Autodesk Inventor part; units mm, degrees
(part 3 of 3)
  line L1481 (57.9743, 33.8467) -> (57.6371, 34.1533)
  line L1482 (57.6371, 34.1533) -> (57.3304, 34.4906)
  line L1483 (57.3304, 34.4906) -> (57.0572, 34.8563)
  line L1484 (57.0572, 34.8563) -> (56.8192, 35.2478)
  line L1485 (56.8192, 35.2478) -> (56.6194, 35.6631)
  line L1486 (56.6194, 35.6631) -> (56.4595, 36.0994)
  line L1487 (56.4595, 36.0994) -> (56.3424, 36.5547)
  line L1488 (56.3424, 36.5547) -> (56.2704, 37.0263)
  line L1489 (56.2704, 37.0263) -> (56.2459, 37.5119)
  line L1490 (-65.7501, 37.5) -> (-65.7256, 37.9856)
  line L1491 (-65.7256, 37.9856) -> (-65.6536, 38.4573)
  line L1492 (-65.6536, 38.4573) -> (-65.5365, 38.9125)
  line L1493 (-65.5365, 38.9125) -> (-65.3768, 39.3488)
  line L1494 (-65.3768, 39.3488) -> (-65.1768, 39.7642)
  line L1495 (-65.1768, 39.7642) -> (-64.9389, 40.1557)
  line L1496 (-64.9389, 40.1557) -> (-64.6654, 40.5214)
  line L1497 (-64.6654, 40.5214) -> (-64.3588, 40.8588)
  line L1498 (-64.3588, 40.8588) -> (-64.0215, 41.1653)
  line L1499 (-64.0215, 41.1653) -> (-63.6558, 41.4388)
  line L1500 (-63.6558, 41.4388) -> (-63.2643, 41.6767)
  line L1501 (-63.2643, 41.6767) -> (-62.849, 41.8767)
  line L1502 (-62.849, 41.8767) -> (-62.4126, 42.0364)
  line L1503 (-62.4126, 42.0364) -> (-61.9574, 42.1535)
  line L1504 (-61.9574, 42.1535) -> (-61.4857, 42.2255)
  line L1505 (-61.4857, 42.2255) -> (-61.0002, 42.25)
  line L1506 (-61.0002, 42.25) -> (-60.5144, 42.2255)
  line L1507 (-60.5144, 42.2255) -> (-60.0428, 42.1535)
  line L1508 (-60.0428, 42.1535) -> (-59.5877, 42.0364)
  line L1509 (-59.5877, 42.0364) -> (-59.1512, 41.8767)
  line L1510 (-59.1512, 41.8767) -> (-58.736, 41.6767)
  line L1511 (-58.736, 41.6767) -> (-58.3443, 41.4388)
  line L1512 (-58.3443, 41.4388) -> (-57.9786, 41.1653)
  line L1513 (-57.9786, 41.1653) -> (-57.6414, 40.8588)
  line L1514 (-57.6414, 40.8588) -> (-57.3347, 40.5214)
  line L1515 (-57.3347, 40.5214) -> (-57.0614, 40.1557)
  line L1516 (-57.0614, 40.1557) -> (-56.8233, 39.7642)
  line L1517 (-56.8233, 39.7642) -> (-56.6233, 39.3488)
  line L1518 (-56.6233, 39.3488) -> (-56.4637, 38.9125)
  line L1519 (-56.4637, 38.9125) -> (-56.3465, 38.4573)
  line L1520 (-56.3465, 38.4573) -> (-56.2747, 37.9856)
  line L1521 (-56.2747, 37.9856) -> (-56.2501, 37.5)
  line L1522 (-56.2501, 37.5) -> (-56.2747, 37.0143)
  line L1523 (-56.2747, 37.0143) -> (-56.3465, 36.5426)
  line L1524 (-56.3465, 36.5426) -> (-56.4637, 36.0875)
  line L1525 (-56.4637, 36.0875) -> (-56.6233, 35.6511)
  line L1526 (-56.6233, 35.6511) -> (-56.8233, 35.2359)
  line L1527 (-56.8233, 35.2359) -> (-57.0614, 34.8442)
  line L1528 (-57.0614, 34.8442) -> (-57.3347, 34.4785)
  line L1529 (-57.3347, 34.4785) -> (-57.6414, 34.1412)
  line L1530 (-57.6414, 34.1412) -> (-57.9786, 33.8346)
  line L1531 (-57.9786, 33.8346) -> (-58.3443, 33.5613)
  line L1532 (-58.3443, 33.5613) -> (-58.736, 33.3234)
  line L1533 (-58.736, 33.3234) -> (-59.1512, 33.1232)
  line L1534 (-59.1512, 33.1232) -> (-59.5877, 32.9635)
  line L1535 (-59.5877, 32.9635) -> (-60.0428, 32.8466)
  line L1536 (-60.0428, 32.8466) -> (-60.5144, 32.7746)
  line L1537 (-60.5144, 32.7746) -> (-61.0002, 32.7499)
  line L1538 (-61.0002, 32.7499) -> (-61.4857, 32.7746)
  line L1539 (-61.4857, 32.7746) -> (-61.9574, 32.8466)
  line L1540 (-61.9574, 32.8466) -> (-62.4126, 32.9635)
  line L1541 (-62.4126, 32.9635) -> (-62.849, 33.1232)
  line L1542 (-62.849, 33.1232) -> (-63.2643, 33.3234)
  line L1543 (-63.2643, 33.3234) -> (-63.6558, 33.5613)
  line L1544 (-63.6558, 33.5613) -> (-64.0215, 33.8346)
  line L1545 (-64.0215, 33.8346) -> (-64.3588, 34.1412)
  line L1546 (-64.3588, 34.1412) -> (-64.6654, 34.4785)
  line L1547 (-64.6654, 34.4785) -> (-64.9389, 34.8442)
  line L1548 (-64.9389, 34.8442) -> (-65.1768, 35.2359)
  line L1549 (-65.1768, 35.2359) -> (-65.3768, 35.6511)
  line L1550 (-65.3768, 35.6511) -> (-65.5365, 36.0875)
  line L1551 (-65.5365, 36.0875) -> (-65.6536, 36.5426)
  line L1552 (-65.6536, 36.5426) -> (-65.7256, 37.0143)
  line L1553 (-65.7256, 37.0143) -> (-65.7501, 37.5)
  line L1554 (58.9, 61.0109) -> (58.9107, 61.2257)
  line L1555 (58.9107, 61.2257) -> (58.9427, 61.4341)
  line L1556 (58.9427, 61.4341) -> (58.9944, 61.6355)
  line L1557 (58.9944, 61.6355) -> (59.065, 61.8284)
  line L1558 (59.065, 61.8284) -> (59.1532, 62.0121)
  line L1559 (59.1532, 62.0121) -> (59.2587, 62.1852)
  line L1560 (59.2587, 62.1852) -> (59.3796, 62.3468)
  line L1561 (59.3796, 62.3468) -> (59.515, 62.4959)
  line L1562 (59.515, 62.4959) -> (59.6641, 62.6315)
  line L1563 (59.6641, 62.6315) -> (59.8257, 62.7524)
  line L1564 (59.8257, 62.7524) -> (59.999, 62.8575)
  line L1565 (59.999, 62.8575) -> (60.1826, 62.946)
  line L1566 (60.1826, 62.946) -> (60.3756, 63.0167)
  line L1567 (60.3756, 63.0167) -> (60.5768, 63.0683)
  line L1568 (60.5768, 63.0683) -> (60.7852, 63.1002)
  line L1569 (60.7852, 63.1002) -> (60.9998, 63.111)
  line L1570 (60.9998, 63.111) -> (61.2148, 63.1002)
  line L1571 (61.2148, 63.1002) -> (61.4232, 63.0683)
  line L1572 (61.4232, 63.0683) -> (61.6244, 63.0167)
  line L1573 (61.6244, 63.0167) -> (61.8173, 62.946)
  line L1574 (61.8173, 62.946) -> (62.001, 62.8575)
  line L1575 (62.001, 62.8575) -> (62.1739, 62.7524)
  line L1576 (62.1739, 62.7524) -> (62.3358, 62.6315)
  line L1577 (62.3358, 62.6315) -> (62.485, 62.4959)
  line L1578 (62.485, 62.4959) -> (62.6204, 62.3468)
  line L1579 (62.6204, 62.3468) -> (62.7413, 62.1852)
  line L1580 (62.7413, 62.1852) -> (62.8464, 62.0121)
  line L1581 (62.8464, 62.0121) -> (62.9349, 61.8284)
  line L1582 (62.9349, 61.8284) -> (63.0055, 61.6355)
  line L1583 (63.0055, 61.6355) -> (63.0572, 61.4341)
  line L1584 (63.0572, 61.4341) -> (63.0889, 61.2257)
  line L1585 (63.0889, 61.2257) -> (63.0999, 61.0109)
  line L1586 (63.0999, 61.0109) -> (63.0889, 60.7963)
  line L1587 (63.0889, 60.7963) -> (63.0572, 60.5879)
  line L1588 (63.0572, 60.5879) -> (63.0055, 60.3865)
  line L1589 (63.0055, 60.3865) -> (62.9349, 60.1936)
  line L1590 (62.9349, 60.1936) -> (62.8464, 60.0099)
  line L1591 (62.8464, 60.0099) -> (62.7413, 59.8368)
  line L1592 (62.7413, 59.8368) -> (62.6204, 59.6753)
  line L1593 (62.6204, 59.6753) -> (62.485, 59.5261)
  line L1594 (62.485, 59.5261) -> (62.3358, 59.3905)
  line L1595 (62.3358, 59.3905) -> (62.1739, 59.2696)
  line L1596 (62.1739, 59.2696) -> (62.001, 59.1645)
  line L1597 (62.001, 59.1645) -> (61.8173, 59.076)
  line L1598 (61.8173, 59.076) -> (61.6244, 59.0054)
  line L1599 (61.6244, 59.0054) -> (61.4232, 58.9537)
  line L1600 (61.4232, 58.9537) -> (61.2148, 58.9218)
  line L1601 (61.2148, 58.9218) -> (60.9998, 58.911)
  line L1602 (60.9998, 58.911) -> (60.7852, 58.9218)
  line L1603 (60.7852, 58.9218) -> (60.5768, 58.9537)
  line L1604 (60.5768, 58.9537) -> (60.3756, 59.0054)
  line L1605 (60.3756, 59.0054) -> (60.1826, 59.076)
  line L1606 (60.1826, 59.076) -> (59.999, 59.1645)
  line L1607 (59.999, 59.1645) -> (59.8257, 59.2696)
  line L1608 (59.8257, 59.2696) -> (59.6641, 59.3905)
  line L1609 (59.6641, 59.3905) -> (59.515, 59.5261)
  line L1610 (59.515, 59.5261) -> (59.3796, 59.6753)
  line L1611 (59.3796, 59.6753) -> (59.2587, 59.8368)
  line L1612 (59.2587, 59.8368) -> (59.1532, 60.0099)
  line L1613 (59.1532, 60.0099) -> (59.065, 60.1936)
  line L1614 (59.065, 60.1936) -> (58.9944, 60.3865)
  line L1615 (58.9944, 60.3865) -> (58.9427, 60.5879)
  line L1616 (58.9427, 60.5879) -> (58.9107, 60.7963)
  line L1617 (58.9107, 60.7963) -> (58.9, 61.0109)
  line L1618 (-63.1006, 61.0109) -> (-63.0898, 61.2257)
  line L1619 (-63.0898, 61.2257) -> (-63.0579, 61.4341)
  line L1620 (-63.0579, 61.4341) -> (-63.0062, 61.6355)
  line L1621 (-63.0062, 61.6355) -> (-62.9356, 61.8284)
  line L1622 (-62.9356, 61.8284) -> (-62.8472, 62.0121)
  line L1623 (-62.8472, 62.0121) -> (-62.742, 62.1852)
  line L1624 (-62.742, 62.1852) -> (-62.6211, 62.3468)
  line L1625 (-62.6211, 62.3468) -> (-62.4855, 62.4959)
  line L1626 (-62.4855, 62.4959) -> (-62.3365, 62.6315)
  line L1627 (-62.3365, 62.6315) -> (-62.1748, 62.7524)
  line L1628 (-62.1748, 62.7524) -> (-62.0016, 62.8575)
  line L1629 (-62.0016, 62.8575) -> (-61.818, 62.946)
  line L1630 (-61.818, 62.946) -> (-61.6251, 63.0167)
  line L1631 (-61.6251, 63.0167) -> (-61.4239, 63.0683)
  line L1632 (-61.4239, 63.0683) -> (-61.2153, 63.1002)
  line L1633 (-61.2153, 63.1002) -> (-61.0007, 63.111)
  line L1634 (-61.0007, 63.111) -> (-60.7859, 63.1002)
  line L1635 (-60.7859, 63.1002) -> (-60.5774, 63.0683)
  line L1636 (-60.5774, 63.0683) -> (-60.3761, 63.0167)
  line L1637 (-60.3761, 63.0167) -> (-60.1831, 62.946)
  line L1638 (-60.1831, 62.946) -> (-59.9997, 62.8575)
  line L1639 (-59.9997, 62.8575) -> (-59.8266, 62.7524)
  line L1640 (-59.8266, 62.7524) -> (-59.6648, 62.6315)
  line L1641 (-59.6648, 62.6315) -> (-59.5157, 62.4959)
  line L1642 (-59.5157, 62.4959) -> (-59.3801, 62.3468)
  line L1643 (-59.3801, 62.3468) -> (-59.2593, 62.1852)
  line L1644 (-59.2593, 62.1852) -> (-59.1541, 62.0121)
  line L1645 (-59.1541, 62.0121) -> (-59.0657, 61.8284)
  line L1646 (-59.0657, 61.8284) -> (-58.9951, 61.6355)
  line L1647 (-58.9951, 61.6355) -> (-58.9433, 61.4341)
  line L1648 (-58.9433, 61.4341) -> (-58.9114, 61.2257)
  line L1649 (-58.9114, 61.2257) -> (-58.9005, 61.0109)
  line L1650 (-58.9005, 61.0109) -> (-58.9114, 60.7963)
  line L1651 (-58.9114, 60.7963) -> (-58.9433, 60.5879)
  line L1652 (-58.9433, 60.5879) -> (-58.9951, 60.3865)
  line L1653 (-58.9951, 60.3865) -> (-59.0657, 60.1936)
  line L1654 (-59.0657, 60.1936) -> (-59.1541, 60.0099)
  line L1655 (-59.1541, 60.0099) -> (-59.2593, 59.8368)
  line L1656 (-59.2593, 59.8368) -> (-59.3801, 59.6753)
  line L1657 (-59.3801, 59.6753) -> (-59.5157, 59.5261)
  line L1658 (-59.5157, 59.5261) -> (-59.6648, 59.3905)
  line L1659 (-59.6648, 59.3905) -> (-59.8266, 59.2696)
  line L1660 (-59.8266, 59.2696) -> (-59.9997, 59.1645)
  line L1661 (-59.9997, 59.1645) -> (-60.1831, 59.076)
  line L1662 (-60.1831, 59.076) -> (-60.3761, 59.0054)
  line L1663 (-60.3761, 59.0054) -> (-60.5774, 58.9537)
  line L1664 (-60.5774, 58.9537) -> (-60.7859, 58.9218)
  line L1665 (-60.7859, 58.9218) -> (-61.0007, 58.911)
  line L1666 (-61.0007, 58.911) -> (-61.2153, 58.9218)
  line L1667 (-61.2153, 58.9218) -> (-61.4239, 58.9537)
  line L1668 (-61.4239, 58.9537) -> (-61.6251, 59.0054)
  line L1669 (-61.6251, 59.0054) -> (-61.818, 59.076)
  line L1670 (-61.818, 59.076) -> (-62.0016, 59.1645)
  line L1671 (-62.0016, 59.1645) -> (-62.1748, 59.2696)
  line L1672 (-62.1748, 59.2696) -> (-62.3365, 59.3905)
  line L1673 (-62.3365, 59.3905) -> (-62.4855, 59.5261)
  line L1674 (-62.4855, 59.5261) -> (-62.6211, 59.6753)
  line L1675 (-62.6211, 59.6753) -> (-62.742, 59.8368)
  line L1676 (-62.742, 59.8368) -> (-62.8472, 60.0099)
  line L1677 (-62.8472, 60.0099) -> (-62.9356, 60.1936)
  line L1678 (-62.9356, 60.1936) -> (-63.0062, 60.3865)
  line L1679 (-63.0062, 60.3865) -> (-63.0579, 60.5879)
  line L1680 (-63.0579, 60.5879) -> (-63.0898, 60.7963)
  line L1681 (-63.0898, 60.7963) -> (-63.1006, 61.0109)
  line L1682 (-63.1006, -60.9971) -> (-63.0898, -60.7825)
  line L1683 (-63.0898, -60.7825) -> (-63.0579, -60.5741)
  line L1684 (-63.0579, -60.5741) -> (-63.0062, -60.3729)
  line L1685 (-63.0062, -60.3729) -> (-62.9356, -60.18)
  line L1686 (-62.9356, -60.18) -> (-62.8472, -59.9963)
  line L1687 (-62.8472, -59.9963) -> (-62.742, -59.823)
  line L1688 (-62.742, -59.823) -> (-62.6211, -59.6615)
  line L1689 (-62.6211, -59.6615) -> (-62.4855, -59.5123)
  line L1690 (-62.4855, -59.5123) -> (-62.3365, -59.3769)
  line L1691 (-62.3365, -59.3769) -> (-62.1748, -59.256)
  line L1692 (-62.1748, -59.256) -> (-62.0016, -59.1509)
  line L1693 (-62.0016, -59.1509) -> (-61.818, -59.0624)
  line L1694 (-61.818, -59.0624) -> (-61.6251, -58.9917)
  line L1695 (-61.6251, -58.9917) -> (-61.4239, -58.9401)
  line L1696 (-61.4239, -58.9401) -> (-61.2153, -58.908)
  line L1697 (-61.2153, -58.908) -> (-61.0007, -58.8974)
  line L1698 (-61.0007, -58.8974) -> (-60.7859, -58.908)
  line L1699 (-60.7859, -58.908) -> (-60.5774, -58.9401)
  line L1700 (-60.5774, -58.9401) -> (-60.3761, -58.9917)
  line L1701 (-60.3761, -58.9917) -> (-60.1831, -59.0624)
  line L1702 (-60.1831, -59.0624) -> (-59.9997, -59.1509)
  line L1703 (-59.9997, -59.1509) -> (-59.8266, -59.256)
  line L1704 (-59.8266, -59.256) -> (-59.6648, -59.3769)
  line L1705 (-59.6648, -59.3769) -> (-59.5157, -59.5123)
  line L1706 (-59.5157, -59.5123) -> (-59.3801, -59.6615)
  line L1707 (-59.3801, -59.6615) -> (-59.2593, -59.823)
  line L1708 (-59.2593, -59.823) -> (-59.1541, -59.9963)
  line L1709 (-59.1541, -59.9963) -> (-59.0657, -60.18)
  line L1710 (-59.0657, -60.18) -> (-58.9951, -60.3729)
  line L1711 (-58.9951, -60.3729) -> (-58.9433, -60.5741)
  line L1712 (-58.9433, -60.5741) -> (-58.9114, -60.7825)
  line L1713 (-58.9114, -60.7825) -> (-58.9005, -60.9971)
  line L1714 (-58.9005, -60.9971) -> (-58.9114, -61.2121)
  line L1715 (-58.9114, -61.2121) -> (-58.9433, -61.4205)
  line L1716 (-58.9433, -61.4205) -> (-58.9951, -61.6217)
  line L1717 (-58.9951, -61.6217) -> (-59.0657, -61.8147)
  line L1718 (-59.0657, -61.8147) -> (-59.1541, -61.9983)
  line L1719 (-59.1541, -61.9983) -> (-59.2593, -62.1716)
  line L1720 (-59.2593, -62.1716) -> (-59.3801, -62.3331)
  line L1721 (-59.3801, -62.3331) -> (-59.5157, -62.4823)
  line L1722 (-59.5157, -62.4823) -> (-59.6648, -62.6177)
  line L1723 (-59.6648, -62.6177) -> (-59.8266, -62.7386)
  line L1724 (-59.8266, -62.7386) -> (-59.9997, -62.8437)
  line L1725 (-59.9997, -62.8437) -> (-60.1831, -62.9322)
  line L1726 (-60.1831, -62.9322) -> (-60.3761, -63.0029)
  line L1727 (-60.3761, -63.0029) -> (-60.5774, -63.0545)
  line L1728 (-60.5774, -63.0545) -> (-60.7859, -63.0866)
  line L1729 (-60.7859, -63.0866) -> (-61.0007, -63.0973)
  line L1730 (-61.0007, -63.0973) -> (-61.2153, -63.0866)
  line L1731 (-61.2153, -63.0866) -> (-61.4239, -63.0545)
  line L1732 (-61.4239, -63.0545) -> (-61.6251, -63.0029)
  line L1733 (-61.6251, -63.0029) -> (-61.818, -62.9322)
  line L1734 (-61.818, -62.9322) -> (-62.0016, -62.8437)
  line L1735 (-62.0016, -62.8437) -> (-62.1748, -62.7386)
  line L1736 (-62.1748, -62.7386) -> (-62.3365, -62.6177)
  line L1737 (-62.3365, -62.6177) -> (-62.4855, -62.4823)
  line L1738 (-62.4855, -62.4823) -> (-62.6211, -62.3331)
  line L1739 (-62.6211, -62.3331) -> (-62.742, -62.1716)
  line L1740 (-62.742, -62.1716) -> (-62.8472, -61.9983)
  line L1741 (-62.8472, -61.9983) -> (-62.9356, -61.8147)
  line L1742 (-62.9356, -61.8147) -> (-63.0062, -61.6217)
  line L1743 (-63.0062, -61.6217) -> (-63.0579, -61.4205)
  line L1744 (-63.0579, -61.4205) -> (-63.0898, -61.2121)
  line L1745 (-63.0898, -61.2121) -> (-63.1006, -60.9971)
  line L1746 (58.9, -60.9971) -> (58.9107, -60.7825)
  line L1747 (58.9107, -60.7825) -> (58.9427, -60.5741)
  line L1748 (58.9427, -60.5741) -> (58.9944, -60.3729)
  line L1749 (58.9944, -60.3729) -> (59.065, -60.18)
  line L1750 (59.065, -60.18) -> (59.1532, -59.9963)
  line L1751 (59.1532, -59.9963) -> (59.2587, -59.823)
  line L1752 (59.2587, -59.823) -> (59.3796, -59.6615)
  line L1753 (59.3796, -59.6615) -> (59.515, -59.5123)
  line L1754 (59.515, -59.5123) -> (59.6641, -59.3769)
  line L1755 (59.6641, -59.3769) -> (59.8257, -59.256)
  line L1756 (59.8257, -59.256) -> (59.999, -59.1509)
  line L1757 (59.999, -59.1509) -> (60.1826, -59.0624)
  line L1758 (60.1826, -59.0624) -> (60.3756, -58.9917)
  line L1759 (60.3756, -58.9917) -> (60.5768, -58.9401)
  line L1760 (60.5768, -58.9401) -> (60.7852, -58.908)
  line L1761 (60.7852, -58.908) -> (60.9998, -58.8974)
  line L1762 (60.9998, -58.8974) -> (61.2148, -58.908)
  line L1763 (61.2148, -58.908) -> (61.4232, -58.9401)
  line L1764 (61.4232, -58.9401) -> (61.6244, -58.9917)
  line L1765 (61.6244, -58.9917) -> (61.8173, -59.0624)
  line L1766 (61.8173, -59.0624) -> (62.001, -59.1509)
  line L1767 (62.001, -59.1509) -> (62.1739, -59.256)
  line L1768 (62.1739, -59.256) -> (62.3358, -59.3769)
  line L1769 (62.3358, -59.3769) -> (62.485, -59.5123)
  line L1770 (62.485, -59.5123) -> (62.6204, -59.6615)
  line L1771 (62.6204, -59.6615) -> (62.7413, -59.823)
  line L1772 (62.7413, -59.823) -> (62.8464, -59.9963)
  line L1773 (62.8464, -59.9963) -> (62.9349, -60.18)
  line L1774 (62.9349, -60.18) -> (63.0055, -60.3729)
  line L1775 (63.0055, -60.3729) -> (63.0572, -60.5741)
  line L1776 (63.0572, -60.5741) -> (63.0889, -60.7825)
  line L1777 (63.0889, -60.7825) -> (63.0999, -60.9971)
  line L1778 (63.0999, -60.9971) -> (63.0889, -61.2121)
  line L1779 (63.0889, -61.2121) -> (63.0572, -61.4205)
  line L1780 (63.0572, -61.4205) -> (63.0055, -61.6217)
  line L1781 (63.0055, -61.6217) -> (62.9349, -61.8147)
  line L1782 (62.9349, -61.8147) -> (62.8464, -61.9983)
  line L1783 (62.8464, -61.9983) -> (62.7413, -62.1716)
  line L1784 (62.7413, -62.1716) -> (62.6204, -62.3331)
  line L1785 (62.6204, -62.3331) -> (62.485, -62.4823)
  line L1786 (62.485, -62.4823) -> (62.3358, -62.6177)
  line L1787 (62.3358, -62.6177) -> (62.1739, -62.7386)
  line L1788 (62.1739, -62.7386) -> (62.001, -62.8437)
  line L1789 (62.001, -62.8437) -> (61.8173, -62.9322)
  line L1790 (61.8173, -62.9322) -> (61.6244, -63.0029)
  line L1791 (61.6244, -63.0029) -> (61.4232, -63.0545)
  line L1792 (61.4232, -63.0545) -> (61.2148, -63.0866)
  line L1793 (61.2148, -63.0866) -> (60.9998, -63.0973)
  line L1794 (60.9998, -63.0973) -> (60.7852, -63.0866)
  line L1795 (60.7852, -63.0866) -> (60.5768, -63.0545)
  line L1796 (60.5768, -63.0545) -> (60.3756, -63.0029)
  line L1797 (60.3756, -63.0029) -> (60.1826, -62.9322)
  line L1798 (60.1826, -62.9322) -> (59.999, -62.8437)
  line L1799 (59.999, -62.8437) -> (59.8257, -62.7386)
  line L1800 (59.8257, -62.7386) -> (59.6641, -62.6177)
  line L1801 (59.6641, -62.6177) -> (59.515, -62.4823)
  line L1802 (59.515, -62.4823) -> (59.3796, -62.3331)
  line L1803 (59.3796, -62.3331) -> (59.2587, -62.1716)
  line L1804 (59.2587, -62.1716) -> (59.1532, -61.9983)
  line L1805 (59.1532, -61.9983) -> (59.065, -61.8147)
  line L1806 (59.065, -61.8147) -> (58.9944, -61.6217)
  line L1807 (58.9944, -61.6217) -> (58.9427, -61.4205)
  line L1808 (58.9427, -61.4205) -> (58.9107, -61.2121)
  line L1809 (58.9107, -61.2121) -> (58.9, -60.9971)
  line L1810 (-107.5002, 0) -> (107.5, 0) construction
  line L1811 (0, -107.5001) -> (0, 107.5001) construction
  point P0 (0, 0)
  point P1 (0, 0)
  constraints: 2964 end point, 5 midpoint, 321 other
sketch "Sketch2" plane through (0, 0, 0) normal (0, 0, 1) x (1, 0, 0)
  line L0 (-107.5002, 101.5001) -> (-107.5002, -101.5001) construction
  line L1 (101.5, 107.5001) -> (-101.5, 107.5001) construction
  line L2 (107.5, -101.5001) -> (107.5, 101.5001) projected
  line L3 (-101.5, -107.5001) -> (101.5, -107.5001) projected
  line L4 (-101.5002, 107.5001) -> (101.5, 107.5001)
  line L5 (107.5, 101.5001) -> (107.5, -101.5001)
  line L6 (101.5, -107.5001) -> (-101.5002, -107.5001)
  line L7 (-107.5002, -101.5001) -> (-107.5002, 101.5001)
  arc A0 (-107.5002, -101.5001) -> (-101.5002, -107.5001) centre (-101.5002, -101.5001) ccw
  arc A1 (101.5, -107.5001) -> (107.5, -101.5001) centre (101.5, -101.5001) ccw
  arc A2 (107.5, 101.5001) -> (101.5, 107.5001) centre (101.5, 101.5001) ccw
  arc A3 (-101.5002, 107.5001) -> (-107.5002, 101.5001) centre (-101.5002, 101.5001) ccw
  line L8 (-82.5268, 97.5093) -> (-8.2921, 97.5093)
  line L9 (-8.2921, 97.5093) -> (-45.4095, 60.3918)
  line L10 (-45.4095, 60.3918) -> (-82.5268, 97.5093)
  line L11 (8.2719, 97.5093) -> (82.4876, 97.5093)
  line L12 (82.4876, 97.5093) -> (45.3797, 60.4015)
  line L13 (45.3797, 60.4015) -> (8.2719, 97.5093)
  line L14 (72.0062, 57.0482) -> (97.4996, 82.5416)
  line L15 (97.4996, 82.5416) -> (97.4996, 3.9999)
  line L16 (97.4996, 3.9999) -> (72.0062, 3.9999)
  line L17 (72.0062, 3.9999) -> (72.0062, 57.0482)
  line L18 (72.0062, -4.0001) -> (97.4996, -4.0001)
  line L19 (97.4996, -4.0001) -> (97.4996, -82.5021)
  line L20 (97.4996, -82.5021) -> (72.0062, -57.0088)
  line L21 (72.0062, -57.0088) -> (72.0062, -4.0001)
  line L22 (50.0062, -35.0087) -> (50.0062, 35.0482)
  line L23 (50.0062, 35.0482) -> (19.4003, 4.4423)
  line L24 (19.4003, 4.4423) -> (19.4003, -4.4028)
  line L25 (19.4003, -4.4028) -> (50.0062, -35.0087)
  line L26 (45.3797, -60.2857) -> (82.4876, -97.3935)
  line L27 (82.4876, -97.3935) -> (8.2719, -97.3935)
  line L28 (8.2719, -97.3935) -> (45.3797, -60.2857)
  line L29 (41.1371, -56.0431) -> (4.0017, -93.1785)
  line L30 (4.0017, -93.1785) -> (4.0017, -18.9081)
  line L31 (4.0017, -18.9081) -> (41.1371, -56.0431)
  line L32 (-3.9981, -18.8647) -> (-3.9981, -93.2022)
  line L33 (-3.9981, -93.2022) -> (-41.1669, -56.0334)
  line L34 (-41.1669, -56.0334) -> (-3.9981, -18.8647)
  line L35 (-45.4095, -60.2761) -> (-82.5268, -97.3935)
  line L36 (-82.5268, -97.3935) -> (-8.2921, -97.3935)
  line L37 (-8.2921, -97.3935) -> (-45.4096, -60.2762)
  line L38 (-97.4892, -82.4901) -> (-72.0064, -57.007)
  line L39 (-72.0064, -57.007) -> (-72.0064, -4.0001)
  line L40 (-72.0064, -4.0001) -> (-97.4892, -4.0001)
  line L41 (-97.4892, -4.0001) -> (-97.4892, -82.4901)
  line L42 (-97.4892, 4.0106) -> (-72.0064, 3.9999)
  line L43 (-72.0064, 3.9999) -> (-72.0064, 57.0089)
  line L44 (-72.0064, 57.0089) -> (-97.4892, 82.4918)
  line L45 (-97.4892, 82.4918) -> (-97.4892, 4.0106)
  line L46 (-50.0063, -35.007) -> (-19.4509, -4.4518)
  line L47 (-19.4509, -4.4518) -> (-19.4509, 4.4535)
  line L48 (-19.4509, 4.4535) -> (-50.0063, 35.0089)
  line L49 (-50.0063, 35.0089) -> (-50.0063, -35.007)
  line L50 (4.0017, 19.0236) -> (41.1371, 56.1588)
  line L51 (41.1371, 56.1588) -> (4.0017, 93.294)
  line L52 (4.0017, 93.294) -> (4.0017, 19.0236)
  line L53 (-41.1669, 56.1492) -> (-3.9981, 93.318)
  line L54 (-3.9981, 93.318) -> (-3.9981, 18.9804)
  line L55 (-3.9981, 18.9804) -> (-41.1669, 56.1492)
  point P0 (0, 0)
  point P1 (82.4876, -97.3935)
  dimension "d0" = 6
  constraints: 104 end point, 19 perpendicular, 15 parallel, 8 point on circle, 8 tangent, 4 centre point, 3 equal radius, 1 collinear, 1 horizontal, 1 point on line
  measures "d0" radius of A0
extrude "Extrusion1" add sketch "Sketch2" along normal blind 2
sketch "Sketch3" plane through (0, 0, 0) normal (0, 0, -1) x (-1, 0, 0)
  line L0 (101.5002, -107.5001) -> (-101.5, -107.5001) projected
  line L1 (107.5002, 101.5001) -> (107.5002, -101.5001) projected
  arc A0 (107.5002, 101.5001) -> (101.5002, 107.5001) centre (101.5002, 101.5001) ccw projected
  line L2 (-101.5, 107.5001) -> (101.5002, 107.5001) projected
  arc A1 (-101.5, 107.5001) -> (-107.5, 101.5001) centre (-101.5, 101.5001) ccw projected
  line L3 (-107.5, -101.5001) -> (-107.5, 101.5001) projected
  circle A2 centre (-100.5, 100.5001) radius 1.6
  line L4 (0.0001, 107.5001) -> (0.0001, -107.5001) construction
  line L5 (-107.5, 0) -> (107.5002, 0) construction
  circle A3 centre (100.5002, 100.5001) radius 1.6
  circle A4 centre (-100.5, -100.5001) radius 1.6
  circle A5 centre (100.5002, -100.5001) radius 1.6
  point P0 (0, 0)
  point P1 (101.5002, 101.5001)
  point P2 (101.5002, -101.5001)
  point P3 (-101.5, -101.5001)
  point P4 (101.5002, -101.5001)
  dimension "d3" = 3.2
  dimension "d4" = 7
  dimension "d5" = 7
  constraints: 7 symmetric about line, 4 centre point, 4 end point, 4 midpoint, 3 other
  measures "d3" diameter of A2
  measures "d4" distance from line of L2 A2.centre
  measures "d5" distance from line of L3 A2.centre
extrude "Extrusion2" cut sketch "Sketch3" against normal through all
body "Solid1"
